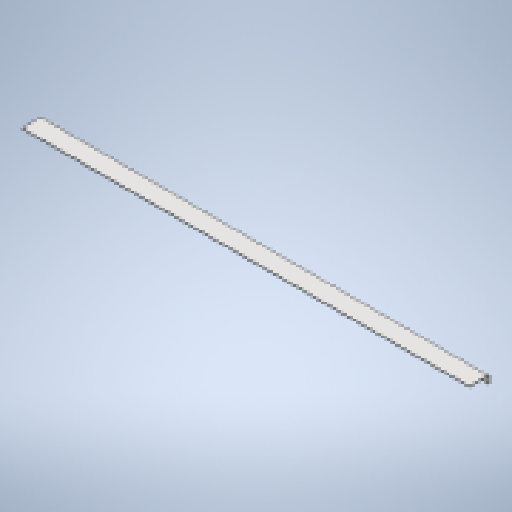
# Autodesk Inventor part: GBK-RK-0043 rib 3
Saved by Autodesk Inventor 2026.2 (Build 302298000, 298)
## iProperties
Created: 2026-09-14
Part Number: GBK-RK-0043 rib 3
Material: Generic
Document SubType Name: Sheet Metal
Designer: admin
Density: 1 g/cm^3
Flat Pattern Width: 6.65239 cm
Flat Pattern Length: 110.4 cm
Flat Pattern Area: 734.424 cm^2
Sheet Metal Rule: Default_mm
Sheet Metal Width: 66,524 mm
Sheet Metal Length: 1104,000 mm
Sheet Metal Area: 73442,378 mm^2
Appearance: Default
Author: admin
Autodesk Inventor part; units mm, degrees
ref_plane "YZ Plane" through (0, 0, 0) normal (1, 0, 0) x (0, 1, 0)
ref_plane "XZ Plane" through (0, 0, 0) normal (0, 1, 0) x (-1, 0, 0)
ref_plane "XY Plane" through (0, 0, 0) normal (0, 0, 1) x (1, 0, 0)
sketch "Sketch3" plane through (0, 0, 0) normal (0, 1, 0) x (-1, 0, 0)
  line L0 (0, 0) -> (-1104, 0)
  line L1 (-1104, 0) -> (-1104, -50)
  line L2 (-1104, -50) -> (0, -50)
  line L3 (0, -50) -> (0, 0)
  dimension "d25" = 50
  dimension "d28" = 1104
  measures "d25" distance of L0.end L1.end
  measures "d28" distance of L0.start L0.end
extrude "Plate3" add sketch "Sketch3" along normal blind 2
sketch "Sketch4" plane through (1104, 2, -48) normal (0, 0, -1) x (-1, 0, 0)
  line L0 (1104, 0) -> (0, 0)
  line L1 (0, 0) -> (0, -20)
  line L2 (0, -20) -> (1104, -20)
  line L3 (1104, -20) -> (1104, 0)
  constraints: 6 end point, 1 horizontal, 1 perpendicular, 1 vertical
edge flange "Flange2" height 20 angle 90 thickness 2 bend radius 2 thickness toward (0, 0, -1) relief tear relief width 2 relief depth 1 edges at (552, 0, -50) wall of the first edge with corners at (0, 2, -48) (1104, 2, -48) (1104, -18, -48) (0, -18, -48)
bend "Bend3"
corner "Corner3"
equation "\"d30\" = Thickness"
equation "\"d31\" = BendReliefWidth"
equation "\"d32\" = BendReliefDepth"
equation "\"d33\" = MinimumRemnant"
equation "\"d34\" = TransitionRadius"
equation "\"d37\" = BendRadius"
equation "\"d38\" = CornerReliefSize"
equation "\"d39\" = GapSize"
equation "\"d40\" = JacobiRadiusSize"
equation "\"BendRadius\" = Thickness"
equation "\"BendReliefWidth\" = Thickness"
equation "\"BendReliefDepth\" = 0.5 * Thickness"
equation "\"CornerReliefSize\" = 4 * Thickness"
equation "\"MinimumRemnant\" = 2 * Thickness"
equation "\"TransitionRadius\" = BendRadius"
equation "\"JacobiRadiusSize\" = BendRadius"
equation "\"GapSize\" = Thickness"
equation "\"Thickness\" = 2"
body "Solid2"
